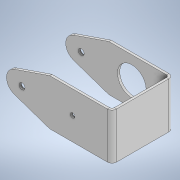
# Autodesk Inventor part: New frame
Saved by Autodesk Inventor 2020 (Build 240168000, 168)
## iProperties
Created: 2022-07-01
Part Number: New frame
Material: Generic
Document SubType Name: Sheet Metal
Designer: karimi2
Density: 1 g/cm^3
Sheet Metal Rule: Default_mm
Appearance: Default
Author: karimi2
Autodesk Inventor part; units mm, degrees
ref_plane "YZ Plane" through (0, 0, 0) normal (1, 0, 0) x (0, 1, 0)
ref_plane "XZ Plane" through (0, 0, 0) normal (0, 1, 0) x (-1, 0, 0)
ref_plane "XY Plane" through (0, 0, 0) normal (0, 0, 1) x (1, 0, 0)
sketch "Sketch1" plane through (0, 0, 0) normal (0, 0, 1) x (1, 0, 0)
  line L0 (77.5, -20) -> (-77.5, -20)
  line L1 (-77.5, 20) -> (77.5, 20)
  line L2 (115, -20) -> (-115, 20) construction
  line L3 (-115, -20) -> (115, 20) construction
  arc A0 (-108.2432, 9.4595) -> (-108.2432, -9.4595) centre (-105, 0) ccw
  line L4 (-25, 20) -> (-25, -20)
  line L5 (0, 20) -> (0, -20) construction
  line L6 (25, 20) -> (25, -20)
  line L7 (-77.5, 20) -> (-77.5, -20) construction
  line L8 (77.5, 20) -> (77.5, -20) construction
  line L9 (-77.5, 20) -> (-108.2432, 9.4595)
  line L10 (-77.5, -20) -> (-108.2432, -9.4595)
  arc A1 (108.2432, -9.4595) -> (108.2432, 9.4595) centre (105, 0) ccw
  line L11 (77.5, 20) -> (108.2432, 9.4595)
  line L12 (77.5, -20) -> (108.2432, -9.4595)
  circle A2 centre (-101.5, 0) radius 2.6
  circle A3 centre (101.5, 0) radius 2.6
  circle A4 centre (57.5, 0) radius 2
  circle A5 centre (-57.5, 0) radius 12.5
  point P0 (0, 0)
  dimension "d0" = 230
  dimension "d1" = 40
  dimension "d2" = 25
  dimension "d3" = 25
  dimension "d6" = 52.5
  dimension "d7" = 52.5
  dimension "d8" = 20
  dimension "d9" = 20
  dimension "d10" = 24
  dimension "d11" = 24
  dimension "d13" = 5.2
  dimension "d14" = 5.2
  dimension "d17" = 32.5
  dimension "d18" = 4
  dimension "d21" = 25
  dimension "d22" = 32.5
  dimension "d23" = 37.849
  dimension "d24" = 71.075
  dimension "d25" = 151.21
  dimension "d26" = 9.059
  dimension "d27" = 88.1081
  dimension "d28" = 44.054
  dimension "d29" = 44.054
  dimension "d30" = 12.1622
  dimension "d31" = 25.6757
  dimension "d32" = 11.1351
  dimension "d33" = 25.4054
  measures "d0" distance of L2.end L3.end
  measures "d1" distance of L3.start L2.end
  measures "d2" distance between parallel lines of L4 L5
  measures "d3" distance between parallel lines of L6 L5
  measures "d6" distance from line of L7 L4.start
  measures "d7" distance between parallel lines of L8 L6
  measures "d8" diameter of A0
  measures "d9" diameter of A1
  measures "d10" distance from line of L7 A2.centre
  measures "d11" distance from line of L8 A3.centre
  measures "d13" diameter of A2
  measures "d14" diameter of A3
  measures "d17" distance from line of L6 A4.centre
  measures "d18" diameter of A4
  measures "d21" diameter of A5
  measures "d22" distance from line of L4 A5.centre
  measures "d23" angle of L11 L12
  measures "d24" angle of L11 L8
  measures "d25" angle of L3 L11
  measures "d26" angle of L2 L11
  measures "d27" distance between parallel lines of L11 L10
  measures "d28" distance from line of point (0, 0) L11
  measures "d29" distance from line of point (0, 0) L12
  measures "d30" distance from line of L3.end L11
  measures "d31" distance from line of L2.start L11
  measures "d32" distance from line of A3.centre L11
  measures "d33" distance from line of A4.centre L11
extrude "Plate1" add sketch "Sketch1" along normal blind 2
sketch "Sketch2" plane through (0, 0, 2) normal (0, 0, 1) x (1, 0, 0)
  line L0 (0, 30.7812) -> (0, -33.2812) construction
  line L1 (-25, 20) -> (-25, -20)
  line L2 (77.5, -20) -> (-77.5, -20) projected
  point P0 (0, 0)
  point P1 (0, -20)
  dimension "d38" = 25
  dimension "d39" = 40
  constraints: 4 end point, 2 vertical, 1 horizontal alignment, 1 midpoint
  measures "d38" distance between parallel lines of L0 L1
  measures "d39" distance of L1.start L1.end
fold "Fold1" angle 90 bend radius 2 thickness 2 k factor 0.44 line from (-25, 20, 2) to (-25, -20, 2) line at bend centre moving side (1, 0, 0) folds toward (0, 0, 1)
sketch "Sketch4" plane through (-23.2619, 0, 131.7381) normal (1, 0, 0) x (0, 0, -1)
  line L0 (80, -20) -> (80, 20)
  line L1 (127.7381, 20) -> (27.5, 20) projected
  point P0 (131.7381, 0)
  dimension "d46" = 52.5
  constraints: 2 end point, 1 point on line, 1 vertical
  measures "d46" distance from line of L0 L1.end
fold "Fold2" angle 90 bend radius 2 thickness 2 k factor 0.44 line from (-23.2619, -20, 51.7381) to (-23.2619, 20, 51.7381) line at bend centre moving side (0, 0, 1) folds toward (-1, 0, 0)
equation "\"d34\" = Thickness"
equation "\"d40\" = BendReliefWidth"
equation "\"d41\" = BendReliefDepth"
equation "\"d42\" = MinimumRemnant"
equation "\"d43\" = TransitionRadius"
equation "\"d45\" = BendRadius"
equation "\"d47\" = BendReliefWidth"
equation "\"d48\" = BendReliefDepth"
equation "\"d49\" = MinimumRemnant"
equation "\"d50\" = TransitionRadius"
equation "\"d52\" = BendRadius"
equation "\"BendRadius\" = Thickness"
equation "\"BendReliefWidth\" = Thickness"
equation "\"BendReliefDepth\" = 0.5 * Thickness"
equation "\"CornerReliefSize\" = 4 * Thickness"
equation "\"MinimumRemnant\" = 2 * Thickness"
equation "\"TransitionRadius\" = BendRadius"
equation "\"JacobiRadiusSize\" = BendRadius"
equation "\"GapSize\" = Thickness"
equation "\"Thickness\" = 2"
body "Solid1"
